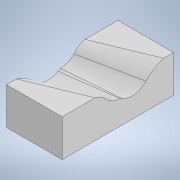
# Autodesk Inventor part: crazy_test_2
Saved by Autodesk Inventor 2021 (Build 250183000, 183)
## iProperties
Created: 2020-10-26
Part Number: crazy_test_2
Material: Generic
Document SubType Name: Modeling
Designer: asandman
Density: 1 g/cm^3
Appearance: Default
Author: asandman
Autodesk Inventor part; units mm, degrees
ref_plane "YZ Plane" through (0, 0, 0) normal (1, 0, 0) x (0, 1, 0)
ref_plane "XZ Plane" through (0, 0, 0) normal (0, 1, 0) x (-1, 0, 0)
ref_plane "XY Plane" through (0, 0, 0) normal (0, 0, 1) x (1, 0, 0)
sketch "Sketch1" plane through (0, 0, 0) normal (0, 1, 0) x (-1, 0, 0)
  line L0 (0, 0) -> (15, 0)
  line L1 (15, 0) -> (15, -30)
  line L2 (15, -30) -> (0, -30)
  line L3 (0, -30) -> (0, 0)
  dimension "d0" = 15
  dimension "d1" = 30
  constraints: 8 end point, 2 parallel, 1 horizontal, 1 perpendicular
  measures "d0" distance of L1.end L2.end
  measures "d1" distance of L0.end L1.end
extrude "Extrusion1" add sketch "Sketch1" along normal blind 10
sketch "Sketch2" plane through (0, 0, 0) normal (1, 0, 0) x (0, 0, -1)
  line L0 (30, 10) -> (0, 10) projected
  arc A0 (11.8554, 8.0947) -> (8.8495, 10) centre (7.6947, 4.8542) ccw
  arc A1 (11.8554, 8.0947) -> (15.4691, 6.5404) centre (15.5119, 11.6182) ccw
  arc A2 (15.4691, 6.5404) -> (16.1182, 6.2019) centre (17.0614, 8.802) ccw
  arc A3 (16.1182, 6.2019) -> (22.5713, 7.0384) centre (18.8148, 10.7083) ccw
  arc A4 (27.3203, 10) -> (22.5713, 7.0384) centre (31.0109, -1.2064) ccw
  line L1 (27.3203, 10) -> (8.8495, 10)
  point P0 (0, 0)
  dimension "d4" = 2.6797
  dimension "d6" = 8.8495
  constraints: 10 point on circle, 5 centre point, 2 end point, 2 point on line, 1 tangent
  measures "d4" distance of L0.start L1.start
  measures "d6" distance of L0.end L1.end
sketch "Sketch4" plane through (-15, 0, -30) normal (-1, 0, 0) x (0, 0, 1)
  line L0 (30, 10) -> (0, 10)
  arc A0 (11.8554, 8.0947) -> (8.8495, 10) centre (7.6947, 4.8542) ccw
  arc A1 (11.8554, 8.0947) -> (15.4691, 6.5404) centre (15.5119, 11.6182) ccw
  arc A2 (15.4691, 6.5404) -> (16.1182, 6.2019) centre (17.0614, 8.802) ccw
  arc A3 (16.1182, 6.2019) -> (22.5713, 7.0384) centre (18.8148, 10.7083) ccw
  arc A4 (27.3203, 10) -> (22.5713, 7.0384) centre (31.0109, -1.2064) ccw
  line L1 (27.3203, 10) -> (8.8495, 10)
  point P0 (30, 0)
  point P1 (0, 0)
  dimension "d8" = 2.6797
  dimension "d9" = 8.8495
  constraints: 10 point on circle, 5 centre point, 4 end point, 2 point on line, 1 tangent
  measures "d8" distance of L0.start L1.start
  measures "d9" distance of L0.end L1.end
loft "Loft1" cut profiles "Sketch2", "Sketch4"
body "Solid1"
